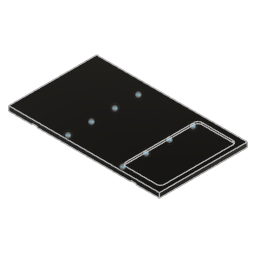
Shelf-Cover (Autodesk Fusion 360 design; units mm, degrees)
Autodesk Fusion 360 part; units mm, degrees
sketch "Sketch3" plane through (0, 0, -6.985) normal (0, 0, -1) x (1, 0, 0)
  line L0 (-175.8934, -9.525) -> (-175.8934, -177.8)
  line L1 (-175.8934, -177.8) -> (-14.6034, -177.8)
  line L2 (-14.6034, -177.8) -> (-14.6034, -9.525)
  line L3 (-14.6034, -9.525) -> (-175.8934, -9.525)
  circle A0 centre (-40.0034, -165.1) radius 0
  line L4 (-27.3034, -147.955) -> (-27.3034, -22.225)
  line L5 (-163.1934, -147.955) -> (-163.1934, -22.225)
  line L6 (-95.2484, 13.4719) -> (-95.2484, -190.0784)
  circle A1 centre (-150.4934, -165.1) radius 0
  circle A2 centre (-40.0034, -117.6867) radius 0
  circle A3 centre (-150.4934, -117.6867) radius 0
  circle A4 centre (-40.0034, -70.2733) radius 0
  circle A5 centre (-150.4934, -70.2733) radius 0
  circle A6 centre (-40.0034, -22.86) radius 0
  circle A7 centre (-150.4934, -22.86) radius 0
  circle A8 centre (-40.0034, -165.1) radius 0
  circle A9 centre (-40.0034, -117.6867) radius 0
  circle A10 centre (-40.0034, -70.2733) radius 0
  circle A11 centre (-40.0034, -22.86) radius 0
  circle A12 centre (-150.4934, -165.1) radius 0
  circle A13 centre (-150.4934, -117.6867) radius 0
  circle A14 centre (-150.4934, -70.2733) radius 0
  circle A15 centre (-150.4934, -22.86) radius 0
  dimension "d1" = 0
  dimension "d2" = 12.7
  dimension "d3" = 12.7
  dimension "d4" = 0
  dimension "d5" = 0
  constraint perpendicular L1 L6
  constraint concentric A0 A8
  constraint concentric A1 A12
  measures "d1" diameter of A0
  measures "d2" horizontal distance of A0.centre L4.start
  measures "d3" distance of L1 A0.centre
  measures "d4" diameter of A8
  measures "d5" diameter of A12
sketch "Sketch1" plane through (0, 0, 0) normal (0, 0, 1) x (-1, 0, 0)
  circle A0 centre (195.2625, -165.1) radius 2.1082
  line L0 (190.5, 0) -> (190.5, -177.8)
  line L1 (190.5, -177.8) -> (200.025, -177.8)
  line L2 (200.025, -177.8) -> (200.025, 0)
  line L3 (200.025, 0) -> (190.5, 0)
  circle A1 centre (-4.7625, -165.1) radius 2.1082
  line L4 (0, -177.8) -> (0, 0)
  line L5 (0, 0) -> (-9.525, 0)
  line L6 (-9.525, 0) -> (-9.525, -177.8)
  line L7 (-9.525, -177.8) -> (0, -177.8)
  line L8 (0, 0) -> (0, -177.8)
  line L9 (0, -88.9) -> (190.5, -88.9)
  line L10 (-57.15, 0) -> (247.65, 0)
  line L11 (247.65, 0) -> (247.65, -177.8)
  line L12 (247.65, -177.8) -> (-57.15, -177.8)
  line L13 (-57.15, -177.8) -> (-57.15, 0)
  line L14 (95.25, 0) -> (95.25, -177.8) construction
  line L15 (247.65, -88.9) -> (-57.15, -88.9) construction
  point P0 (95.25, -88.9)
  point P1 (95.25, -88.9)
  dimension "d61" = 304.8
  dimension "d62" = 177.8
  constraint midpoint L8 L9.start
  constraint midpoint L0 L9.end
  constraint horizontal L10
  constraint vertical L11
  constraint horizontal L12
  constraint vertical L13
  constraint midpoint L10 L14.start
  constraint midpoint L12 L14.end
  constraint midpoint L11 L15.start
  constraint midpoint L13 L15.end
  constraint midpoint L14 P1
  constraint midpoint L9 P1
  constraint coincident P1 P0
  measures "d61" distance of L10.start L10.end
  measures "d62" distance of L10.start L12.end
extrude "Extrude1" add sketch "Sketch1" along normal blind 7.62 contours A0 | L0 L1 L2 L3 L10 L12 | L0 L4 L8 L9 L10 | L0 L4 L8 L9 L12 | L2 L10 L11 L12 | L4 L5 L6 L7 L8 L10 L12 | L6 L10 L12 L13 | A1
extrude "Extrude2" add sketch "Sketch1" against normal blind 1.905 contours L0 L4 L8 L9 L10 | L0 L4 L8 L9 L12 | L2 L10 L11 L12 | L6 L10 L12 L13
move_face "OffsetFaces1" offset -0.1 4 faces at (9.525, 59.2667, -0.635) (0, 118.5333, -0.635) (-200.025, 59.2667, -1.27) (-190.5, 118.5333, -1.27)
sketch "Sketch2" plane through (0, 0, 7.62) normal (0, 0, 1) x (-1, 0, 0)
  line L0 (-57.15, -177.8) -> (247.65, -177.8)
  line L1 (247.65, -177.8) -> (247.65, 0)
  line L2 (247.65, 0) -> (-57.15, 0)
  line L3 (-57.15, 0) -> (-57.15, -177.8)
  line L4 (23.005, -11.7729) -> (-40.005, -11.7729)
  line L5 (-47.625, -19.3929) -> (-47.625, -158.4029)
  line L6 (-40.005, -166.0229) -> (23.005, -166.0229)
  line L7 (30.625, -158.4029) -> (30.625, -19.3929)
  arc A0 (-40.005, -11.7729) -> (-47.625, -19.3929) centre (-40.005, -19.3929) ccw
  arc A1 (-47.625, -158.4029) -> (-40.005, -166.0229) centre (-40.005, -158.4029) ccw
  arc A2 (23.005, -166.0229) -> (30.625, -158.4029) centre (23.005, -158.4029) ccw
  arc A3 (30.625, -19.3929) -> (23.005, -11.7729) centre (23.005, -19.3929) ccw
  point P0 (30.625, -11.7729)
  point P1 (-47.625, -11.7729)
  point P2 (30.625, -166.0229)
  dimension "d114" = 154.25
  dimension "d115" = 78.25
  dimension "d117" = 11.7729
  dimension "d118" = 11.7771
  dimension "d119" = 7.62
  dimension "d133" = 9.525
  constraint horizontal L4
  constraint vertical L5
  constraint horizontal L6
  constraint vertical L7
  constraint coincident P1 L4
  constraint coincident P1 L5
  constraint tangent L4 A0
  constraint tangent L5 A0
  constraint tangent L5 A1
  constraint tangent L6 A1
  constraint equal A0 A1
  constraint coincident P2 L6
  constraint coincident P2 L7
  constraint tangent L6 A2
  constraint tangent L7 A2
  constraint equal A0 A2
  constraint coincident P0 L7
  constraint coincident P0 L4
  constraint tangent L7 A3
  constraint tangent L4 A3
  constraint equal A0 A3
  measures "d114" distance of P0 P2
  measures "d115" distance of P0 P1
  measures "d117" distance of L2 L4
  measures "d118" distance of L0 L6
  measures "d119" radius of A0
  measures "d133" distance of L3 L5
extrude "Extrude4" cut sketch "Sketch2" against normal blind 3.81 contours L4 L5 L6 L7 A0 A1 A2 A3
sketch "sketch 1030" plane through (0, 0, -6.985) normal (0, 0, -1) x (1, 0, 0)
  circle A0 centre (-150.4934, -117.6867) radius 2.1082
  circle A1 centre (-150.4934, -22.86) radius 2.1082
  circle A2 centre (-40.0034, -70.2733) radius 2.1082
  circle A3 centre (-40.0034, -165.1) radius 2.1082
  circle A4 centre (-40.0034, -117.6867) radius 2.1082
  circle A5 centre (-40.0034, -22.86) radius 2.1082
  circle A6 centre (-150.4934, -70.2733) radius 2.1082
  circle A7 centre (-150.4934, -165.1) radius 2.1082
extrude "Extrude5" cut sketch "sketch 1030" against normal blind 10
equation "d1 = M4ScrewClearenceFit"
equation "d4 = M4HeadDiameter"
equation "d5 = M4HeadDiameter"
